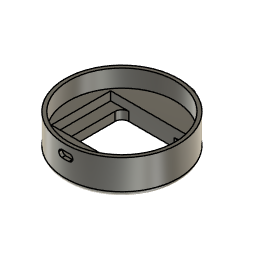
HackCharmCase v7 (Autodesk Fusion 360 design; units mm, degrees)
Autodesk Fusion 360 part; units mm, degrees
sketch "Sketch1" plane through (0, 0, 0) normal (0, 0, 1) x (1, 0, 0)
  line L0 (23.5, 17) -> (-23.5, 17)
  line L1 (-23.5, 17) -> (-23.5, -17)
  line L2 (-23.5, -17) -> (23.5, -17)
  line L3 (23.5, -17) -> (23.5, 17)
  line L4 (23.5, 17) -> (-23.5, -17) construction
  line L5 (-23.5, 17) -> (23.5, -17) construction
  circle A0 centre (0, 0) radius 32.5
  line L6 (7.35, -5.317) -> (-7.35, 5.317) construction
  line L7 (-6.8031, -4.9214) -> (7.35, 5.317) construction
  line L8 (17, -17) -> (-17, -17)
  line L9 (-17, -17) -> (-17, 17)
  line L10 (-17, 17) -> (17, 17)
  line L11 (17, 17) -> (17, -17)
  line L12 (17, -17) -> (-17, 17) construction
  line L13 (-17, -17) -> (17, 17) construction
  circle A1 centre (0, 0) radius 30.5
  circle A2 centre (0, 32.5) radius 5
  circle A3 centre (0, 32.5) radius 7
  dimension "d3" = 47
  dimension "d4" = 34
  dimension "d5" = 65
  dimension "d7" = 34
  dimension "d8" = 34
  dimension "d15" = -2
  dimension "d21" = 10
  dimension "d22" = 2
  constraint horizontal L0
  constraint perpendicular L0 L1
  constraint coincident L4 A0.centre
  constraint coincident L5 A0.centre
  constraint coincident A0.centre A1.centre
  constraint coincident L6 A0.centre
  constraint coincident L7 A0.centre
  constraint coincident L5 L6.start
  constraint horizontal L8
  constraint perpendicular L8 L9
  constraint parallel L8 L10
  constraint parallel L9 L11
  constraint coincident L12 A0.centre
  constraint coincident L13 A0.centre
  constraint coincident A0 A2.centre
  measures "d3" distance of L1.end L2.end
  measures "d4" distance of L0.end L1.end
  measures "d5" diameter of A0
  measures "d7" distance of L9.end L10.end
  measures "d8" distance of L8.end L9.end
  measures "d21" diameter of A2
extrude "Extrude1" add sketch "Sketch1" against normal blind 10 contours L0 L2 L3 L11 | L0 L1 L2 L9 | A0 A1 A3 | A0 A1 A2 A3 | A0 A1 A2 A3 | A0 A1 A2 | A1 A2 A3 | A1 A3 | A1 A2
extrude "Extrude2" cut sketch "Sketch1" against normal blind 5 contours L0 L2 L3 L11 | L0 L1 L2 L9
extrude "Extrude3" add sketch "Sketch1" along normal blind 10 contours A0 A1 A3 | A0 A1 A2 A3 | A0 A1 A2 A3 | A0 A1 A2
sketch "Sketch4" plane through (0, 0, 0) normal (0, 1, 0) x (1, 0, 0)
  line L0 (4.0636, -2.283) -> (-3.9364, -2.283)
  line L1 (-3.9364, -2.283) -> (-3.9364, -6.3356)
  line L2 (-3.9364, -6.3356) -> (4.0636, -6.3356)
  line L3 (4.0636, -6.3356) -> (4.0636, -2.283)
  line L4 (4.0636, -2.283) -> (-3.9364, -6.3356) construction
  line L5 (-3.9364, -2.283) -> (4.0636, -6.3356) construction
  point P0 (0.0636, -4.3093)
  dimension "d29" = 8
  constraint horizontal L0
  constraint perpendicular L0 L1
  constraint parallel L0 L2
  constraint parallel L1 L3
  constraint coincident L4 P0
  constraint coincident L5 P0
  constraint midpoint L4 P0
  measures "d29" distance of L0.start L0.end
extrude "Extrude6" add sketch "Sketch1" along normal mid plane 6 contours A0 A2 A3
extrude "Extrude4" cut sketch "Sketch4" along normal blind 10 from the near side of the face at (0.8102, 32.4899, 5.3333)
fillet "Fillet2" radius 3 1 edges at (-30.3006, 11.7525, -10)
fillet "Fillet3" radius 1 2 faces at (0, 38.8209, -3) (0, 38.8209, 3)
fillet "Fillet4" radius 2 4 edges at (-3.9364, -31.2528, 6.3356) (4.0636, -31.2365, 6.3356) (4.0636, -31.2365, 2.283) (-3.9364, -31.2528, 2.283)
fillet "Fillet5" radius 4 4 edges at (17, 17, -7.5) (-17, 17, -7.5) (17, -17, -7.5) (-17, -17, -7.5)
extrude "Extrude5" [suppressed]
sketch "Sketch2" plane through (0, 0, 0) normal (1, 0, 0) x (0, 1, 0)
fillet "Fillet1" [suppressed]
equation "mainDiamater = 50 mm"
equation "screenWidth = 34 mm"
